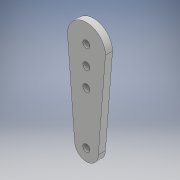
# Autodesk Inventor part: manivela
Saved by Autodesk Inventor 2018 (Build 220112000, 112)
## iProperties
Created: 2020-03-10
Part Number: manivela
Material: Genérico
Document SubType Name: Modeling
Designer: sala.ceri
Density: 1 g/cm^3
Appearance: Valor por defecto
Author: sala.ceri
Autodesk Inventor part; units mm, degrees
ref_plane "YZ Plane" through (0, 0, 0) normal (1, 0, 0) x (0, 1, 0)
ref_plane "XZ Plane" through (0, 0, 0) normal (0, 1, 0) x (-1, 0, 0)
ref_plane "XY Plane" through (0, 0, 0) normal (0, 0, 1) x (1, 0, 0)
sketch "Boceto1" plane through (0, 0, 0) normal (0, 1, 0) x (-1, 0, 0)
  arc A0 (56.9996, -30) -> (66.9996, -30) centre (61.9996, -30) ccw
  circle A1 centre (62, 0) radius 1.5
  circle A2 centre (61.9996, 8) radius 1.5
  circle A3 centre (62, -8) radius 1.5
  line L0 (69.9996, 8) -> (66.9996, -30)
  line L1 (53.9996, 8) -> (56.9996, -30)
  arc A4 (69.9996, 8) -> (53.9996, 8) centre (61.9996, 8) ccw
  circle A5 centre (61.9996, -30) radius 1.5
  dimension "d126" = 3
  constraints: 6 centre point, 4 end point, 4 point on circle, 2 coincident
  measures "d126" diameter of A5
extrude "Extrusión1" add sketch "Boceto1" along normal blind 3
